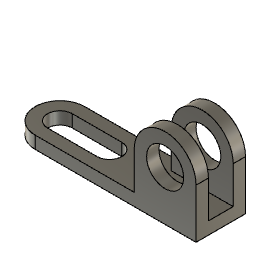
Ex05 (Autodesk Fusion 360 design; units mm, degrees)
Autodesk Fusion 360 part; units mm, degrees
note: some values were not read from the file. Set by a fixed rule: which sketch regions a step uses.
sketch "Sketch1" plane through (0, 0, 0) normal (0, 0, 1) x (1, 0, 0)
  circle A0 centre (0, 0) radius 20
  line L0 (0, 20) -> (130, 20)
  line L1 (130, 20) -> (130, -20)
  line L2 (130, -20) -> (0, -20)
  circle A1 centre (0, 0) radius 10
  line L3 (-33.7231, -17.2923) -> (-73.7231, -17.2923)
  line L4 (0, 0) -> (40, 0) construction
  circle A2 centre (40, 0) radius 10
  line L5 (0, 10) -> (40, 10)
  line L6 (40, -10) -> (0, -10)
  dimension "d1" = 40
  dimension "d2" = 130
  dimension "d3" = 40
  dimension "d4" = 20
  dimension "d6" = 40
  constraint coincident A0.centre A1.centre
  constraint horizontal L0
  constraint vertical L1
  constraint horizontal L2
  constraint coincident A0 L0.start
  constraint horizontal L3
  constraint parallel L0 L4
  constraint coincident L4.end A2.centre
  constraint equal A1 A2
  constraint coincident A1 L5.start
  constraint coincident A2 L5.end
  constraint tangent A2 L5
  constraint parallel L4 L5
  constraint coincident A2 L6.start
  constraint coincident A1 L6.end
  constraint tangent A1 L6
  constraint parallel L5 L6
  measures "d1" diameter of A0
  measures "d2" distance of L1.end L2.end
  measures "d3" distance of L0.end L1.end
  measures "d4" diameter of A1
  measures "d6" distance of A0.centre L4.end
extrude "Extrude1" add sketch "Sketch1" along normal blind 10 contours A0 A1 L5 L6 | A0 L0 L1 L2 A2 L5 L6 picked at (-10.5572, 12.8388)
sketch "Sketch2" plane through (0, -20, 0) normal (0, -1, 0) x (1, 0, 0)
  line L0 (0, 0) -> (130, 0)
  line L1 (130, 0) -> (130, 10)
  line L2 (130, 10) -> (0, 10)
  line L3 (0, 10) -> (0, 0)
  line L4 (80, 10) -> (130, 10)
  line L5 (130, 10) -> (130, 40)
  line L6 (130, 40) -> (80, 40)
  line L7 (80, 40) -> (80, 10)
  circle A0 centre (105, 40) radius 25
  circle A1 centre (105, 40) radius 15
  dimension "d9" = 30
  dimension "d10" = 50
  dimension "d11" = 30
  constraint horizontal L4
  constraint vertical L5
  constraint horizontal L6
  constraint vertical L7
  constraint coincident L2 L4.start
  constraint midpoint L6 A0.centre
  constraint coincident L5.end A0
  constraint concentric A0 A1
  measures "d9" distance of L4.start L6.end
  measures "d10" distance of L5.end L6.end
  measures "d11" diameter of A1
extrude "Extrude2" add sketch "Sketch2" against normal blind 10 contours L2 L4 L5 L7 A0 | L6 A0 A1 | L6 A0 A1
mirror "Mirror1" about plane through (0, 0, 0) normal (0, 1, 0) of "Extrude2"
equation "d4 = ( 10 * 2 ) * 1 mm"
